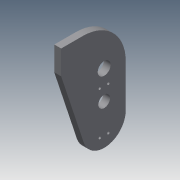
# Autodesk Inventor part: packa_strana(a)
Saved by Autodesk Inventor 2013 (Build 170138000, 138)
## iProperties
Created: 2013-05-25
Part Number: packa_strana(a)
Material: Generic
Document SubType Name: Modeling
Designer: idle-rug
Density: 1 g/cm^3
Author: idle-rug
Autodesk Inventor part; units mm, degrees
ref_plane "YZ Plane" through (0, 0, 0) normal (1, 0, 0) x (0, 1, 0)
ref_plane "XZ Plane" through (0, 0, 0) normal (0, 1, 0) x (-1, 0, 0)
ref_plane "XY Plane" through (0, 0, 0) normal (0, 0, 1) x (1, 0, 0)
sketch "Sketch1" plane through (0, 0, 0) normal (1, 0, 0) x (0, 1, 0)
  circle A0 centre (0, 0) radius 16.575
  line L0 (0, 16.575) -> (0, -49.725)
  line L1 (0, -33.15) -> (0, -15.05)
  line L2 (0, -15.05) -> (0, -70.05)
  line L3 (10, -70.05) -> (-10, -70.05)
  line L4 (-10, -70.05) -> (-10, -15.05)
  line L5 (-10, -15.05) -> (10, -15.05)
  line L6 (10, -15.05) -> (10, -70.05)
  line L7 (10, -70.05) -> (-10, -15.05) construction
  line L8 (-10, -70.05) -> (10, -15.05) construction
  line L9 (10, -62.65) -> (-10, -62.65)
  line L10 (-10, -62.65) -> (-10, -22.45)
  line L11 (-10, -22.45) -> (10, -22.45)
  line L12 (10, -22.45) -> (10, -62.65)
  line L13 (10, -62.65) -> (-10, -22.45) construction
  line L14 (-10, -62.65) -> (10, -22.45) construction
  line L15 (-4.95, -27.2) -> (-4.95, -17.7)
  line L16 (-4.95, -17.7) -> (4.95, -17.7)
  line L17 (4.95, -27.2) -> (-4.95, -17.7) construction
  line L18 (-4.95, -27.2) -> (4.95, -17.7) construction
  line L19 (4.95, -67.4) -> (-4.95, -67.4)
  line L20 (-4.95, -67.4) -> (-4.95, -57.9)
  line L21 (-4.95, -57.9) -> (4.95, -57.9)
  line L22 (4.95, -67.4) -> (-4.95, -57.9) construction
  line L23 (-4.95, -67.4) -> (4.95, -57.9) construction
  circle A1 centre (4.95, -17.7) radius 1.5
  circle A2 centre (-4.95, -17.7) radius 1.5
  circle A3 centre (4.95, -67.4) radius 1.5
  circle A4 centre (-4.95, -67.4) radius 1.5
  circle A5 centre (0, -33.15) radius 6.8
  line L24 (0, -80) -> (0, -55)
  arc A6 (-25, -55) -> (25, -55) centre (0, -55) ccw
  line L25 (0, 0) -> (0, 45)
  line L26 (25, 45) -> (-25, 45)
  line L27 (25, 45) -> (25, -55)
  line L28 (-25, 45) -> (-25, -55)
  circle A7 centre (0, 0) radius 7.5
  point P0 (0, -42.55)
  point P1 (0, -42.55)
  point P2 (0, -22.45)
  point P3 (0, -62.65)
  dimension "d0" = 33.15
  dimension "d2" = 66.3
  dimension "d4" = 18.1
  dimension "d5" = 55
  dimension "d6" = 20
  dimension "d7" = 55
  dimension "d8" = 40.2
  dimension "d9" = 9.9
  dimension "d10" = 9.5
  dimension "d11" = 9.9
  dimension "d12" = 9.5
  dimension "d13" = 3
  dimension "d14" = 3
  dimension "d15" = 3
  dimension "d16" = 3
  dimension "d17" = 13.6
  dimension "d20" = 25
  dimension "d21" = 45
  dimension "d22" = 15
  constraints: 58 end point, 12 midpoint, 7 centre point, 7 coincident, 6 parallel, 6 point on line, 4 perpendicular, 3 horizontal, 2 point on circle, 2 tangent, 1 vertical, 1 vertical alignment, 2 other
  measures "d2" distance of L0.start L0.end
  measures "d4" distance of L1.start L1.end
  measures "d5" distance of L1.end L2.end
  measures "d6" distance of L4.end L5.end
  measures "d7" distance of L3.end L4.end
  measures "d8" distance of L9.end L10.end
  measures "d9" distance of L15.end L16.end
  measures "d10" distance of L15.start L15.end
  measures "d11" distance of L20.end L21.end
  measures "d12" distance of L19.end L20.end
  measures "d13" diameter of A1
  measures "d14" diameter of A2
  measures "d15" diameter of A3
  measures "d16" diameter of A4
  measures "d17" diameter of A5
  measures "d20" distance of L24.start L24.end
  measures "d21" distance of L25.start L25.end
  measures "d22" diameter of A7
extrude "Extrusion1" add sketch "Sketch1" along normal blind 5 contours A0 L5 L0 A7 | A0 L25 L26 L27 A6 L24 L3 L6 L5 | L0 A7 L5 A0 | A0 L5 L4 L3 L24 A6 L28 L26 L25 | L5 L6 L11 L0 A0 | A0 L0 L5 | L5 L0 A0 | A0 L0 L16 A2 L15 L11 L4 L5 | L0 L11 L15 A2 L16 | L6 L9 L2 L0 A5 L11 | L11 L0 A5 L2 L21 L20 L9 L4 | L6 L3 L2 L9 | L9 L20 A4 L19 L2 L3 L4 | L9 L20 L21 L2 | L2 L19 A4 L20 L9
sketch "Sketch2" plane through (0, 0, 0) normal (-1, 0, 0) x (0, 0, 1)
  line L0 (45, 25) -> (45, -25) projected
  line L1 (-55, 25) -> (45, 25) projected
  line L2 (45, 25) -> (-5, 25)
  line L3 (45, 25) -> (45, -25)
  arc A0 (45, -25) -> (-5, 25) centre (-5, -25) ccw
  constraints: 4 end point, 2 point on circle, 2 tangent, 1 centre point, 1 collinear, 1 midpoint
extrude "Extrusion2" cut sketch "Sketch2" against normal blind 5
sketch "Sketch3" plane through (0, 0, 0) normal (-1, 0, 0) x (0, 0, 1)
  arc A0 (45, -25) -> (-5, 25) centre (-5, -25) ccw projected
  arc A1 (-55, 25) -> (-55, -25) centre (-55, 0) ccw projected
  line L0 (45, -25) -> (-55, -25) projected
  line L1 (45, -25) -> (45, -50)
  line L2 (45, -50) -> (17, -50)
  line L3 (17, -50) -> (-62.8113, -23.7483)
  line L4 (45, -25) -> (-55, -25)
  arc A2 (-62.8113, -23.7483) -> (-55, -25) centre (-55, 0) ccw
  dimension "d27" = 25
  dimension "d28" = 28
  constraints: 8 end point, 4 point on circle, 3 tangent, 2 perpendicular, 1 centre point, 1 collinear, 1 concentric
  measures "d27" distance of L0.start L1.end
  measures "d28" distance of L1.end L2.end
extrude "Extrusion3" add sketch "Sketch3" against normal blind 5
sketch "Sketch4" plane through (0, 0, 0) normal (-1, 0, 0) x (0, 0, 1)
  circle A0 centre (0, 0) radius 7.5 projected
  arc A1 (45, -25) -> (-5, 25) centre (-5, -25) ccw projected
  line L0 (-55, 25) -> (-5, 25) projected
  arc A2 (-55, 25) -> (-62.8113, -23.7483) centre (-55, 0) ccw projected
  line L1 (-62.8113, -23.7483) -> (17, -50) projected
  line L2 (17, -50) -> (45, -50) projected
  line L3 (45, -50) -> (45, -25) projected
  circle A3 centre (-33.15, 0) radius 6.8 projected
  circle A4 centre (-67.4, -4.95) radius 1.5 projected
  circle A5 centre (-67.4, 4.95) radius 1.5 projected
  circle A6 centre (-17.7, -4.95) radius 1.5 projected
  circle A7 centre (-17.7, 4.95) radius 1.5 projected
extrude "Extrusion4" add sketch "Sketch4" along normal blind 3
sketch "Sketch5" plane through (-3, 0, 0) normal (-1, 0, 0) x (0, 0, 1)
  circle A0 centre (-33.15, 0) radius 6.8 projected
  circle A1 centre (-17.7, -4.95) radius 1.5 projected
  circle A2 centre (-67.4, 4.95) radius 1.5 projected
  line L0 (-67.4, 4.95) -> (-17.7, 4.95)
  line L1 (-17.7, 4.95) -> (-17.7, -4.95)
  line L2 (-17.7, -4.95) -> (-67.4, -4.95)
  line L3 (-67.4, -4.95) -> (-67.4, 4.95)
  line L4 (-67.4, 0) -> (-17.7, 0)
  line L5 (-22.3, 10) -> (-62.8, 10)
  line L6 (-62.8, 10) -> (-62.8, -10)
  line L7 (-62.8, -10) -> (-22.3, -10)
  line L8 (-22.3, -10) -> (-22.3, 10)
  line L9 (-22.3, 10) -> (-62.8, -10) construction
  line L10 (-62.8, 10) -> (-22.3, -10) construction
  point P0 (-42.55, 0)
  dimension "d33" = 40.5
  dimension "d34" = 20
  constraints: 22 end point, 5 midpoint, 4 parallel, 2 horizontal, 2 perpendicular
  measures "d33" distance of L7.end L6.end
  measures "d34" distance of L6.end L5.end
extrude "Extrusion5" cut sketch "Sketch5" against normal blind 3 contours L4 L8 L2 A0 | A0 L0 L8 L4 | A0 L0 L6 L5 L8 | L2 L8 L7 L6 A0 | L4 L6 L0 A0 | A0 L2 L6 L4
sketch "Sketch6" plane through (0, 0, 0) normal (-1, 0, 0) x (0, 0, 1)
  circle A0 centre (-33.15, 0) radius 6.8 projected
  line L0 (-62.8, 10) -> (-22.3, 10) projected
  line L1 (-62.8, -10) -> (-62.8, 10) projected
  line L2 (-22.3, -10) -> (-62.8, -10) projected
  line L3 (-22.3, 10) -> (-22.3, -10) projected
  point P0 (0, 0)
extrude "Extrusion6" cut sketch "Sketch6" against normal blind 1
sketch "Sketch7" plane through (-3, 0, 0) normal (-1, 0, 0) x (0, 0, 1)
  circle A0 centre (0, 0) radius 7.5 projected
  circle A1 centre (0, 0) radius 5
  dimension "d39" = 10
  constraints: 1 centre point, 1 coincident
  measures "d39" diameter of A1
extrude "Extrusion7" add sketch "Sketch7" against normal blind 3
body "Solid1"
